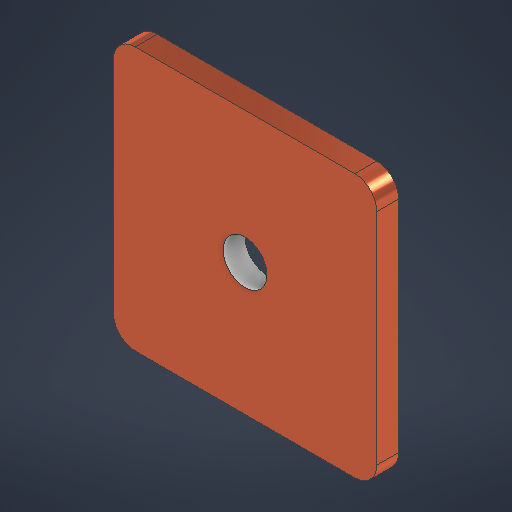
# Autodesk Inventor part: Part1Grroundfinal
Saved by Autodesk Inventor 2026 (Build 300175050, 175E)
## iProperties
Created: 2026-05-06
Part Number: Part1Grroundfinal
Material: Generic
Document SubType Name: Modeling
Designer: ptp527
Density: 1 g/cm^3
Appearance: Default
Author: ptp527
Autodesk Inventor part; units mm, degrees
ref_plane "YZ Plane" through (0, 0, 0) normal (1, 0, 0) x (0, 1, 0)
ref_plane "XZ Plane" through (0, 0, 0) normal (0, 1, 0) x (-1, 0, 0)
ref_plane "XY Plane" through (0, 0, 0) normal (0, 0, 1) x (1, 0, 0)
sketch "Sketch1" plane through (0, 0, 0) normal (0, 0, 1) x (1, 0, 0)
  line L0 (0, 0) -> (600, 0)
  line L1 (600, 0) -> (600, 600)
  line L2 (600, 600) -> (0, 600)
  line L3 (0, 600) -> (0, 0)
  circle A0 centre (300, 300) radius 50
  dimension "d0" = 600
  dimension "d1" = 600
  dimension "d5" = 100
  constraints: 8 end point, 2 parallel, 1 centre point, 1 horizontal, 1 perpendicular
  measures "d0" distance of L1.end L2.end
  measures "d1" distance of L0.end L1.end
  measures "d5" diameter of A0
extrude "Extrusion1" add sketch "Sketch1" along normal blind 50 contours L3 L2 L1 L0 | A0
fillet "Fillet1" radius 50 4 edges at (0, 600, 25) (600, 600, 25) (600, 0, 25) (0, 0, 25)
sketch "Sketch2" plane through (0, 0, 50) normal (0, 0, 1) x (1, 0, 0)
  circle A0 centre (300, 300) radius 50
  line L0 (50, 0) -> (550, 0) projected
  line L1 (550, 600) -> (50, 600) projected
  line L2 (600, 50) -> (600, 550) projected
  point P0 (0, 0)
  point P1 (300, 0)
  dimension "d6" = 100
  dimension "d7" = 300
  dimension "d8" = 300
  dimension "d9" = 300
  constraints: 1 centre point, 1 midpoint
  measures "d6" diameter of A0
  measures "d7" distance of point (300, 0) A0.centre
  measures "d8" distance from line of L1 A0.centre
  measures "d9" distance from line of L2 A0.centre
extrude "Extrusion2" cut sketch "Sketch2" against normal through all
body "Solid1"
